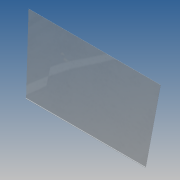
# Autodesk Inventor part: screenInt
Saved by Autodesk Inventor 2013 SP2 (Build 170200200, 200)
## iProperties
Created: 2013-12-16
Part Number: screenInt
Material: Glass
Document SubType Name: Modeling
Designer: Dave
Mass: 98383.3 g
Surface Area: 143280 cm^2
Volume: 45130 cm^3
Density: 2.18 g/cm^3
Author: Dave
Autodesk Inventor part; units mm, degrees
ref_plane "YZ Plane" through (0, 0, 0) normal (1, 0, 0) x (0, 1, 0)
ref_plane "XZ Plane" through (0, 0, 0) normal (0, 1, 0) x (-1, 0, 0)
ref_plane "XY Plane" through (0, 0, 0) normal (0, 0, 1) x (1, 0, 0)
sketch "Sketch1" plane through (0, 0, 0) normal (0, 1, 0) x (-1, 0, 0)
  line L0 (0, 0) -> (-3454.4, 0)
  line L1 (-3454.4, 0) -> (-3454.4, -25.4)
  line L2 (-3454.4, -25.4) -> (0, -25.4)
  line L3 (0, -25.4) -> (0, 0)
  dimension "d0" = 3454.4
  dimension "d1" = 25.4
  constraints: 8 end point, 2 parallel, 1 horizontal, 1 perpendicular
  measures "d0" distance of L0.start L0.end
  measures "d1" distance of L2.end L0.start
extrude "Extrusion1" add sketch "Sketch1" along normal blind 6.35
ref_plane "Work Plane1" through (3454.4, 6.35, -25.4) normal (0, 0.9925462, -0.1218693) x (-1, 0, 0)
sketch "Sketch2" plane through (3454.4, 6.35, -25.4) normal (0, 0.9925462, -0.1218693) x (-1, 0, 0)
  line L0 (0, 6.35) -> (3454.4, 6.35)
  line L1 (3454.4, 6.35) -> (3454.4, 0)
  line L2 (3454.4, 0) -> (0, 0)
  line L3 (0, 0) -> (0, 6.35)
  point P0 (3454.4, 24.4368)
  dimension "d5" = 3454.4
  dimension "d6" = 6.35
  constraints: 8 end point, 2 parallel, 1 horizontal, 1 perpendicular
  measures "d5" distance of L1.end L2.end
  measures "d6" distance of L0.end L1.end
extrude "Extrusion2" add sketch "Sketch2" along normal blind 2032
sketch "Sketch3" plane through (0, 7.1239, -19.0973) normal (0, 0.1218693, 0.9925462) x (1, 0, 0)
  line L0 (3454.4, 2032) -> (3632.2, 2032)
  line L1 (3632.2, 2032) -> (3454.4, 0)
  line L2 (0, 2032) -> (-177.8, 2032)
  line L3 (-177.8, 2032) -> (0, -9.3981)
  line L4 (0, -9.3981) -> (0, 2032)
  line L5 (3454.4, 2032) -> (3454.4, 0)
  dimension "d9" = 177.8
  dimension "d10" = 177.8
  constraints: 12 end point, 1 collinear, 1 parallel, 1 perpendicular
  measures "d9" distance of L0.start L0.end
  measures "d10" distance of L2.start L2.end
extrude "Extrusion3" add sketch "Sketch3" against normal blind 6.35 contours L4 L3 L2
sketch "Sketch4" plane through (0, 7.1239, -19.0973) normal (0, 0.1218693, 0.9925462) x (1, 0, 0)
  line L0 (3454.4, 0) -> (3454.4, 2032) projected
  line L1 (0, -0.7797) -> (0, 0) projected
  line L2 (3454.4, 2032) -> (3632.2, 2032)
  line L3 (3632.2, 2032) -> (3454.4, 0)
  line L4 (3454.4, 2032) -> (3454.4, 0)
  dimension "d13" = 177.8
  constraints: 6 end point, 1 collinear, 1 perpendicular
  measures "d13" distance of L0.end L2.end
extrude "Extrusion4" add sketch "Sketch4" against normal blind 6.35
body "Solid1"
